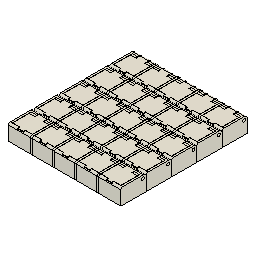
smd-box (Autodesk Fusion 360 design; units mm, degrees)
Autodesk Fusion 360 part; units mm, degrees
note: some values were not read from the file. Set by a fixed rule: which face or edge a step refers to.
sketch "Sketch1" plane through (0, 0, 0) normal (0, 1, 0) x (1, 0, 0) in component "Box"
  line L0 (0, 0) -> (18, 0)
  line L1 (18, 0) -> (18, -19)
  line L2 (18, -19) -> (0, -19)
  line L3 (0, -19) -> (0, 0)
  dimension "d6" = 18
  dimension "d7" = 19
  constraint horizontal L0
  constraint vertical L1
  constraint horizontal L2
  constraint vertical L3
  constraint coincident L0.start L3.end
  measures "d6" distance of L0.start L0.end
  measures "d7" distance of L0.start L2.end
extrude "Extrude1" add sketch "Sketch1" along normal blind 12 makes body 1 in component "Box"
shell "Shell1" thickness 1.4 removed faces 1 at (6, 12, 6.3333) on bodies 1 in component "Box"
copy_body "CutPasteBodies1" bodies 1 removing the originals makes body 2 in component "Box"
sketch "Sketch1 (1)" plane through (0, 12, 0) normal (0, 1, 0) x (-1, 0, 0) in component "Box"
  line L0 (-1.4, 17.6) -> (-1.4, 1.4)
  line L1 (-1.4, 1.4) -> (-16.6, 1.4)
  line L2 (-16.6, 1.4) -> (-16.6, 17.6)
  line L3 (-16.6, 17.6) -> (-1.4, 17.6)
  line L4 (0, 19) -> (-18, 19)
  line L5 (-18, 19) -> (-18, 0)
  line L6 (-18, 0) -> (0, 0)
  line L7 (0, 0) -> (0, 19)
  line L8 (0, 0) -> (-18, 0)
  line L9 (-18, 0) -> (-18, 4.9)
  line L10 (-18, 4.9) -> (0, 4.9)
  line L11 (0, 4.9) -> (0, 0)
  dimension "d13" = 18
  dimension "d14" = 4.9
  constraint horizontal L8
  constraint vertical L9
  constraint horizontal L10
  constraint vertical L11
  constraint coincident L6.end L7.start
  measures "d13" distance of L6.end L5.end
  measures "d14" distance of L6.end L10.end
extrude "Extrude1'" add sketch "Sketch1 (1)" against normal up to surface (10.6 mm away) contours L0 L1 L2 L10 bodies 2 in component "Box"
sketch "Sketch3" plane through (0, 12, 0) normal (0, 1, 0) x (-1, 0, 0) in component "Box"
  line L0 (-1.4, 17.6) -> (-1.4, 4.9)
  line L1 (-1.4, 4.9) -> (-16.6, 4.9)
  line L2 (-16.6, 4.9) -> (-16.6, 17.6)
  line L3 (-16.6, 17.6) -> (-1.4, 17.6)
  line L4 (0, 19) -> (-18, 19)
  line L5 (-18, 19) -> (-18, 0)
  line L6 (-18, 0) -> (0, 0)
  line L7 (0, 0) -> (0, 19)
  line L8 (-9, 0) -> (-9, 4.9) construction
  line L9 (-12.4, 4.9) -> (-5.6, 4.9)
  line L10 (-5.6, 4.9) -> (-5.6, 0)
  line L11 (-5.6, 0) -> (-12.4, 0)
  line L12 (-12.4, 0) -> (-12.4, 4.9)
  line L13 (-12.4, 4.9) -> (-5.6, 0) construction
  line L14 (-5.6, 4.9) -> (-12.4, 0) construction
  point P0 (-9, 2.45)
  dimension "d17" = 6.8
  dimension "d18" = 4.9
  constraint midpoint L6 L8.start
  constraint midpoint L1 L8.end
  constraint perpendicular L9 L10
  constraint parallel L9 L11
  constraint parallel L10 L12
  constraint horizontal L9
  constraint coincident L13 P0
  constraint coincident L14 P0
  constraint midpoint L8 P0
  measures "d17" distance of L10.end L11.end
  measures "d18" distance of L9.end L10.end
extrude "Extrude2" cut sketch "Sketch3" against normal blind 4.9 contours L1 L6 L9 L10 L11 L12 bodies 2 in component "Box"
sketch "Sketch4" plane through (5.6, 0, 0) normal (1, 0, 0) x (0, 0, -1) in component "Box"
  line L0 (0, 12) -> (-4.9, 12)
  line L1 (-4.9, 12) -> (-4.9, 7.1)
  line L2 (-4.9, 7.1) -> (0, 7.1)
  line L3 (0, 7.1) -> (0, 12)
  line L4 (-2.45, 12) -> (-2.45, 7.1) construction
  circle A0 centre (-2.45, 9.55) radius 1.05
  dimension "d21" = 2.1
  constraint midpoint L0 L4.start
  constraint midpoint L2 L4.end
  constraint midpoint L4 A0.centre
  measures "d21" diameter of A0
extrude "Extrude3" cut sketch "Sketch4" along normal up to surface (-5.6 mm away) and the other way up to surface (-12.4 mm away) contours A0 bodies 2 in component "Box"
sketch "Sketch5" plane through (0, 12, 0) normal (0, 1, 0) x (-1, 0, 0) in component "Box"
  line L0 (-5.6, 4.9) -> (-5.6, 0)
  line L1 (-5.6, 0) -> (0, 0)
  line L2 (0, 0) -> (0, 19)
  line L3 (0, 19) -> (-18, 19)
  line L4 (-18, 19) -> (-18, 0)
  line L5 (-18, 0) -> (-12.4, 0)
  line L6 (-12.4, 0) -> (-12.4, 4.9)
  line L7 (-12.4, 4.9) -> (-16.6, 4.9)
  line L8 (-16.6, 4.9) -> (-16.6, 17.6)
  line L9 (-16.6, 17.6) -> (-1.4, 17.6)
  line L10 (-1.4, 17.6) -> (-1.4, 4.9)
  line L11 (-1.4, 4.9) -> (-5.6, 4.9)
  line L12 (-9, 19) -> (-9, 17.6) construction
  line L13 (-11.25, 19) -> (-6.75, 19)
  line L14 (-6.75, 19) -> (-6.75, 17.6)
  line L15 (-6.75, 17.6) -> (-11.25, 17.6)
  line L16 (-11.25, 17.6) -> (-11.25, 19)
  line L17 (-11.25, 19) -> (-6.75, 17.6) construction
  line L18 (-6.75, 19) -> (-11.25, 17.6) construction
  point P0 (-9, 18.3)
  dimension "d29" = 4.5
  dimension "d30" = 1.4
  constraint midpoint L3 L12.start
  constraint midpoint L9 L12.end
  constraint perpendicular L13 L14
  constraint parallel L13 L15
  constraint parallel L14 L16
  constraint horizontal L13
  constraint coincident L17 P0
  constraint coincident L18 P0
  constraint midpoint L12 P0
  measures "d29" distance of L14.end L15.end
  measures "d30" distance of L13.end L14.end
extrude "Extrude4" cut sketch "Sketch5" against normal blind 1.4 contours L3 L9 L13 L14 L15 L16 bodies 2 in component "Box"
ref_plane "WorkPlane1" through (5.78, 9.55, 2.45) normal (1, 0, 0) x (0, 0, 1) in component "Lid"
ref_plane "WorkPlane2" through (12.22, 9.55, 2.45) normal (-1, 0, 0) x (0, 0, -1) in component "Lid"
sketch "Sketch1 (2)" plane through (5.78, 9.725, 2.275) normal (1, 0, 0) x (0, 0, -1) in component "Lid"
  circle A0 centre (-0.175, -0.175) radius 1.05
  line L0 (2.275, 2.275) -> (-2.625, 2.275)
  line L1 (-2.625, 2.275) -> (-2.625, -2.625)
  line L2 (-2.625, -2.625) -> (2.275, -2.625)
  line L3 (2.275, -2.625) -> (2.275, 2.275)
extrude "Extrude1''" add sketch "Sketch1 (2)" along normal up to surface (6.44 mm away) separate body makes body 3 in component "Lid"
extrude "Extrude2'" cut 1 faces at (7.9267, 7.1, 3.2667) along direction (0, 1, 0) blind 0.12 on bodies 3 bodies 3 in component "Lid"
fillet "Fillet1" radius 2.1 1 edges at (9, 7.22, 0) on bodies 3 in component "Lid"
sketch "Sketch2" plane through (0, 12, 0) normal (0, 1, 0) x (-1, 0, 0) in component "Lid"
  line L0 (-12.22, 4.9) -> (-12.22, 0)
  line L1 (-12.22, 0) -> (-5.78, 0)
  line L2 (-5.78, 0) -> (-5.78, 4.9)
  line L3 (-5.78, 4.9) -> (-12.22, 4.9)
  line L4 (-16.6, 4.9) -> (-1.4, 4.9)
  line L5 (-1.4, 4.9) -> (-1.4, 17.6)
  line L6 (-1.4, 17.6) -> (-16.6, 17.6)
  line L7 (-16.6, 17.6) -> (-16.6, 4.9)
extrude "Extrude3'" add sketch "Sketch2" against normal blind 2.1 contours L3 L4 L5 L6 L7 bodies 3 in component "Lid"
extrude "Extrude4'" cut 1 faces at (6.4667, 11.3, 17.6) along direction (0, 0, -1) blind 0.12 on bodies 3 bodies 3 in component "Lid"
extrude "Extrude5" cut 2 faces at (15.14, 11.3, 4.9) (4.32, 11.3, 4.9) along direction (0, 0, 1) blind 0.12 on bodies 3 bodies 3 in component "Lid"
extrude "Extrude6" cut 1 faces at (1.4, 11.3, 9.1733) along direction (1, 0, 0) blind 0.18 on bodies 3 bodies 3 in component "Lid"
extrude "Extrude7" cut 1 faces at (16.6, 10.6, 13.3267) along direction (-1, 0, 0) blind 0.18 on bodies 3 bodies 3 in component "Lid"
sketch "Sketch3 (2)" plane through (0, 0, 17.48) normal (0, 0, 1) x (1, 0, 0) in component "Lid"
  line L0 (16.42, 9.9) -> (16.42, 12)
  line L1 (16.42, 12) -> (1.58, 12)
  line L2 (1.58, 12) -> (1.58, 9.9)
  line L3 (1.58, 9.9) -> (16.42, 9.9)
  line L4 (6.75, 10.6) -> (6.75, 12)
  line L5 (11.25, 10.6) -> (6.75, 10.6)
  line L6 (11.25, 12) -> (11.25, 10.6)
extrude "Extrude8" add sketch "Sketch3 (2)" along normal blind 1.52 contours L1 L4 L5 L6 bodies 3 in component "Lid"
extrude "Extrude9" cut 1 faces at (11.25, 11.5333, 17.9867) along direction (-1, 0, 0) blind 0.18 on bodies 3 bodies 3 in component "Lid"
extrude "Extrude10" cut 1 faces at (6.75, 11.0667, 17.9867) along direction (1, 0, 0) blind 0.18 on bodies 3 bodies 3 in component "Lid"
chamfer "Chamfer1" distance 0.9333 angle 45 1 edges at (9, 10.6, 19) on bodies 3 in component "Lid"
fillet "Fillet2" radius 2.1 1 edges at (9, 12, 0) on bodies 3 in component "Lid"
fillet "Fillet1'" radius 1.4 2 edges at (14.5, 12, 4.9) (3.5, 12, 4.9) on bodies 2 in component "Box"
fillet "Fillet4" radius 1.4 2 edges at (3.68, 9.9, 5.02) (14.32, 9.9, 5.02) on bodies 3 in component "Lid"
fillet "Fillet2'" radius 2.1 2 edges at (15.2, 12, 0) (2.8, 12, 0) on bodies 2 in component "Box"
fillet "Fillet6" radius 1.4 1 edges at (9, 7.22, 4.9) on bodies 3 in component "Lid"
chamfer "Chamfer3" distance 0.7 angle 45 1 edges at (9, 9.9, 4.9) on bodies 3 in component "Lid"
sketch "Sketch4 (2)" plane through (0, 9.9, 0) normal (0, -1, 0) x (1, 0, 0) in component "Lid"
  line L0 (12.22, 5.6) -> (12.22, 6.42)
  line L1 (12.22, 6.42) -> (16.42, 6.42)
  line L2 (16.42, 6.42) -> (16.42, 17.48)
  line L3 (16.42, 17.48) -> (1.58, 17.48)
  line L4 (1.58, 17.48) -> (1.58, 6.42)
  line L5 (1.58, 6.42) -> (5.78, 6.42)
  line L6 (5.78, 6.42) -> (5.78, 5.6)
  line L7 (11.07, 17.48) -> (6.93, 17.48)
  line L8 (11.07, 17.48) -> (11.07, 16.78) construction
  line L9 (6.93, 17.48) -> (11.07, 17.48)
  line L10 (11.07, 17.48) -> (11.07, 16.78)
  line L11 (11.07, 16.78) -> (6.93, 16.78)
  line L12 (6.93, 16.78) -> (6.93, 17.48)
  line L13 (5.78, 5.6) -> (12.22, 5.6)
  dimension "d110" = 0.7
  constraint vertical L8
  constraint coincident L7.start L8.start
  constraint horizontal L9
  constraint vertical L10
  constraint horizontal L11
  constraint vertical L12
  constraint coincident L7.end L9.start
  measures "d110" distance of L7.start L8.end
extrude "Extrude12" add sketch "Sketch4 (2)" along normal blind 1.4 contours L3 L7 L9 L10 L11 L12 bodies 3 in component "Lid"
sketch "Sketch5 (2)" plane through (0, 0, 17.48) normal (0, 0, 1) x (1, 0, 0) in component "Lid"
  line L0 (6.93, 12) -> (1.58, 12)
  line L1 (1.58, 12) -> (1.58, 9.9)
  line L2 (1.58, 9.9) -> (6.93, 9.9)
  line L3 (6.93, 9.9) -> (6.93, 8.5)
  line L4 (6.93, 8.5) -> (11.07, 8.5)
  line L5 (11.07, 8.5) -> (11.07, 9.9)
  line L6 (11.07, 9.9) -> (16.42, 9.9)
  line L7 (16.42, 9.9) -> (16.42, 12)
  line L8 (16.42, 12) -> (11.07, 12)
  line L9 (11.07, 12) -> (11.07, 10.6)
  line L10 (11.07, 10.6) -> (6.93, 10.6)
  line L11 (6.93, 10.6) -> (6.93, 12)
  line L12 (6.93, 8.5) -> (11.07, 8.5)
  line L13 (11.07, 8.5) -> (11.07, 9.2)
  line L14 (11.07, 9.2) -> (6.93, 9.2)
  line L15 (6.93, 9.2) -> (6.93, 8.5)
  constraint horizontal L12
  constraint vertical L13
  constraint horizontal L14
  constraint vertical L15
  constraint midpoint L5 L13.end
  constraint coincident L3.end L4.start
extrude "Extrude13" add sketch "Sketch5 (2)" along normal blind 0.2333 contours L3 L4 L5 L12 L13 L14 L15 bodies 3 in component "Lid"
sketch "Sketch6" plane through (0, 0, 17.6) normal (0, 0, -1) x (-1, 0, 0) in component "Box"
  line L0 (-11.25, 10.6) -> (-11.25, 12)
  line L1 (-11.25, 12) -> (-16.6, 12)
  line L2 (-16.6, 12) -> (-16.6, 1.4)
  line L3 (-16.6, 1.4) -> (-1.4, 1.4)
  line L4 (-1.4, 1.4) -> (-1.4, 12)
  line L5 (-1.4, 12) -> (-6.75, 12)
  line L6 (-6.75, 12) -> (-6.75, 10.6)
  line L7 (-6.75, 10.6) -> (-11.25, 10.6)
  line L8 (-6.93, 9.2) -> (-6.93, 8.5)
  line L9 (-6.93, 8.5) -> (-11.07, 8.5)
  line L10 (-11.07, 8.5) -> (-11.07, 9.2)
  line L11 (-11.07, 9.2) -> (-6.93, 9.2)
extrude "Extrude5'" cut sketch "Sketch6" against normal blind 0.35 contours L8 L9 L10 L11 bodies 2 in component "Box"
fillet "Fillet7" radius 0.21 1 edges at (9, 8.5, 17.7133) on bodies 3 in component "Lid"
chamfer "Chamfer6" distance 1.4 angle 45 1 edges at (9, 9.9, 16.78) on bodies 3 in component "Lid"
fillet "Fillet3" radius 0.21 2 edges at (9, 8.5, 17.95) (9, 9.2, 17.95) on bodies 2 in component "Box"
chamfer "Chamfer2" distance 0.35 angle 45 1 edges at (9, 10.6, 17.6) on bodies 2 in component "Box"
fillet "Fillet4'" radius 1.4 2 edges at (3.375, 12, 19) (14.625, 12, 19) on bodies 2 in component "Box"
pattern_linear "R-Pattern2" count 5 spacing 16.6 along (1, 0, 0) count 5 spacing 19 along (0, 0, 1) of bodies 2 makes body 4 at (22.6, 0, 6.3333) makes body 5 at (39.2, 0, 6.3333) makes body 6 at (55.8, 0, 6.3333) makes body 7 at (72.4, 0, 6.3333) makes body 8 at (6, 0, 25.3333) makes body 9 at (22.6, 0, 25.3333) makes body 10 at (39.2, 0, 25.3333) makes body 11 at (55.8, 0, 25.3333) makes body 12 at (72.4, 0, 25.3333) makes body 13 at (6, 0, 44.3333) makes body 14 at (22.6, 0, 44.3333) makes body 15 at (39.2, 0, 44.3333) makes body 16 at (55.8, 0, 44.3333) makes body 17 at (72.4, 0, 44.3333) makes body 18 at (6, 0, 69.6667) makes body 19 at (22.6, 0, 63.3333) makes body 20 at (39.2, 0, 63.3333) makes body 21 at (55.8, 0, 63.3333) makes body 22 at (72.4, 0, 63.3333) makes body 23 at (6, 0, 88.6667) makes body 24 at (22.6, 0, 82.3333) makes body 25 at (39.2, 0, 82.3333) makes body 26 at (55.8, 0, 82.3333) makes body 27 at (72.4, 0, 82.3333) in component "Box"
pattern_linear "R-Pattern1" count 5 spacing 19 along (0, 0, 1) count 5 spacing 16.6 along (1, 0, 0) of bodies 3 makes body 28 at (26.29, 12, 9.1733) makes body 29 at (41.51, 12, 9.1733) makes body 30 at (58.11, 12, 9.1733) makes body 31 at (74.71, 12, 9.1733) makes body 32 at (9.69, 12, 28.1733) makes body 33 at (8.31, 12, 47.1733) makes body 34 at (8.31, 12, 66.1733) makes body 35 at (9.69, 12, 85.1733) makes body 36 at (26.29, 12, 28.1733) makes body 37 at (26.29, 12, 47.1733) makes body 38 at (24.91, 12, 66.1733) makes body 39 at (26.29, 12, 85.1733) makes body 40 at (41.51, 12, 28.1733) makes body 41 at (42.89, 12, 47.1733) makes body 42 at (41.51, 12, 66.1733) makes body 43 at (41.51, 12, 85.1733) makes body 44 at (58.11, 12, 28.1733) makes body 45 at (59.49, 12, 47.1733) makes body 46 at (58.11, 12, 66.1733) makes body 47 at (58.11, 12, 85.1733) makes body 48 at (74.71, 12, 28.1733) makes body 49 at (74.71, 12, 47.1733) makes body 50 at (74.71, 12, 66.1733) makes body 51 at (74.71, 12, 85.1733) in component "Lid"
component "Box" placed x (1, 0, 0) y (0, 1, 0) z (0, 0, 1) at (0, 0, 0)
component "Lid" placed x (1, 0, 0) y (0, 1, 0) z (0, 0, 1) at (0, 0, 0)
equation "cellWidth = 18 mm"
equation "cellLength = 19 mm"
equation "cellHeight = 12 mm"
equation "d6 = cellWidth"
equation "d7 = cellLength"
equation "d8 = cellHeight"
equation "wallThickness = 1.4 mm"
equation "d11 = wallThickness"
equation "d13 = cellWidth"
equation "d14 = wallThickness * 2 + holeDiam"
equation "d17 = cellWidth - wallThickness * 8"
equation "d18 = wallThickness * 2 + holeDiam"
equation "d19 = -( wallThickness * 2 + holeDiam )"
equation "d21 = holeDiam"
equation "d29 = cellWidth / 4"
equation "d30 = wallThickness"
equation "d31 = -wallThickness"
equation "tolerance = 0.01"
equation "d34 = cellWidth * tolerance"
equation "d35 = cellWidth * tolerance"
equation "d38 = -cellHeight * tolerance"
equation "d40 = holeDiam"
equation "d41 = -wallThickness * 1.5"
equation "d43 = -cellHeight * tolerance"
equation "d45 = -cellHeight * tolerance"
equation "d47 = -cellWidth * tolerance"
equation "d49 = -cellWidth * tolerance"
equation "d51 = wallThickness + cellHeight * tolerance"
equation "d53 = -cellWidth * tolerance"
equation "d55 = -cellWidth * tolerance"
equation "d57 = wallThickness / 1.5"
equation "d78 = holeDiam"
equation "d81 = wallThickness"
equation "d98 = -cellWidth * tolerance"
equation "d101 = wallThickness"
equation "d105 = holeDiam"
equation "d106 = wallThickness"
equation "d107 = wallThickness * 0.5"
equation "d110 = wallThickness * 0.5"
equation "d111 = wallThickness"
equation "d113 = wallThickness / 6"
equation "d115 = -wallThickness * 0.25"
equation "d117 = wallThickness * 0.15"
equation "d119 = wallThickness"
equation "d120 = wallThickness * 0.15"
equation "cellsX = 5"
equation "d127 = cellsX"
equation "d128 = cellsY"
equation "d129 = cellWidth - wallThickness"
equation "d130 = cellLength"
equation "cellsY = 5"
equation "d132 = cellsY"
equation "d133 = cellsX"
equation "d134 = cellLength"
equation "d135 = cellWidth - wallThickness"
equation "holeDiam = 2.1 mm"
equation "d138 = wallThickness / 4"
equation "d139 = wallThickness"
named bodies: "Box", "Box (1)", "Box (2)", "Box (3)", "Box (4)", "Box (8)", "Box (9)", "Box (10)", "Box (11)", "Box (12)", "Box (16)", "Box (17)", "Box (18)", "Box (19)", "Box (20)", "Box (24)", "Box (25)", "Box (26)", "Box (27)", "Box (28)", "Box (32)", "Box (33)", "Box (34)", "Box (35)", "Box (36)"
